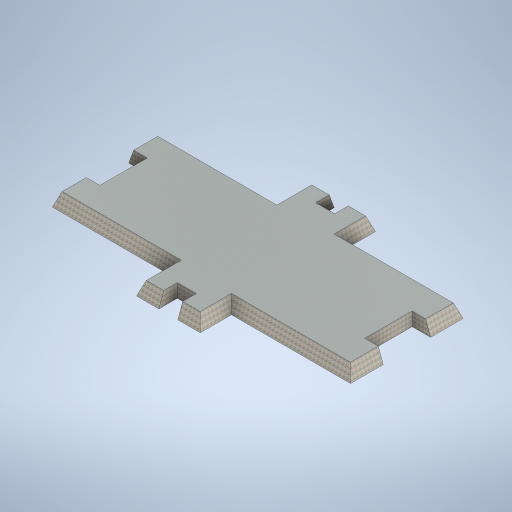
# Autodesk Inventor part: main_floor
Saved by Autodesk Inventor 2024.2 (Build 282272000, 272)
## iProperties
Created: 2024-05-24
Part Number: main_floor
Material: Limestone
Document SubType Name: Modeling
Designer: LOSTER_1
Density: 2.6 g/cm^3
Appearance: Limestone - Ashlar Coursed
Author: LOSTER_1
Autodesk Inventor part; units mm, degrees
ref_plane "YZ Plane" through (0, 0, 0) normal (1, 0, 0) x (0, 1, 0)
ref_plane "XZ Plane" through (0, 0, 0) normal (0, 1, 0) x (-1, 0, 0)
ref_plane "XY Plane" through (0, 0, 0) normal (0, 0, 1) x (1, 0, 0)
sketch "Sketch1" plane through (0, 0, 0) normal (0, 1, 0) x (-1, 0, 0)
  line L0 (-18589.1353, 7057.2083) -> (-18589.1353, -7090.0785)
  line L1 (18609.9901, -7090.0785) -> (18609.9901, 7057.2083)
  line L2 (18609.9901, 7057.2083) -> (21609.9901, 7057.2083)
  line L3 (21609.9901, 7057.2083) -> (21609.9901, -7090.0785)
  line L4 (21609.9901, -7090.0785) -> (18609.9901, -7090.0785)
  line L5 (18609.9901, -7090.0785) -> (18609.9901, 7057.2083)
  line L6 (-18589.1353, 7057.2083) -> (-21589.1353, 7057.2083)
  line L7 (-21589.1353, 7057.2083) -> (-21589.1353, -7090.0785)
  line L8 (-21589.1353, -7090.0785) -> (-18589.1353, -7090.0785)
  line L9 (-18589.1353, -7090.0785) -> (-18589.1353, 7057.2083)
  line L10 (18609.9901, 7057.2083) -> (3994.5778, 7057.2083)
  line L11 (-3973.723, 7057.2083) -> (-18589.1353, 7057.2083)
  line L12 (-18589.1353, -7090.0785) -> (-3973.723, -7090.0785)
  line L13 (3994.5778, -7090.0785) -> (18609.9901, -7090.0785)
  line L14 (3994.5778, -11251.4689) -> (3994.5778, -12251.4689)
  line L15 (3994.5778, -12251.4689) -> (1994.5778, -12251.4689)
  line L16 (-3973.723, 11218.7168) -> (-3973.723, 12218.7168)
  line L17 (-3973.723, 12218.7168) -> (-1973.723, 12218.7168)
  line L18 (3994.5778, -12251.4689) -> (-3973.723, -12251.4689)
  line L19 (-3973.723, -12251.4689) -> (-3973.723, 12218.7168)
  line L20 (-3973.723, 12218.7168) -> (3994.5778, 12218.7168)
  line L21 (3994.5778, 12218.7168) -> (3994.5778, -12251.4689)
  line L22 (21589.1353, 7600) -> (-21589.1353, 7600)
  line L23 (-21589.1353, 7600) -> (-21589.1353, -7600)
  line L24 (-21589.1353, -7600) -> (21589.1353, -7600)
  line L25 (21589.1353, 7600) -> (-21589.1353, -7600) construction
  line L26 (-21589.1353, 7600) -> (21589.1353, -7600) construction
  line L27 (10.4274, -12251.4689) -> (1410.4274, -12251.4689)
  line L28 (1410.4274, -12251.4689) -> (1410.4274, -10251.4689)
  line L29 (1410.4274, -10251.4689) -> (-1389.5726, -10251.4689)
  line L30 (-1389.5726, -10251.4689) -> (-1389.5726, -12251.4689)
  line L31 (10.4274, 12218.7168) -> (1410.4274, 12218.7168)
  line L32 (1410.4274, 12218.7168) -> (1410.4274, 10218.7168)
  line L33 (1410.4274, 10218.7168) -> (-1389.5726, 10218.7168)
  line L34 (-1389.5726, 10218.7168) -> (-1389.5726, 12218.7168)
  line L35 (-21589.1353, 0) -> (-19589.1353, 0)
  line L36 (-19589.1353, 0) -> (-21589.1353, 0)
  line L37 (-21589.1353, 0) -> (-21589.1353, 3500)
  line L38 (21589.1353, 7057.2083) -> (21589.1353, 7600)
  line L39 (21609.9901, -7090.0785) -> (21609.9901, -7600)
  line L40 (21589.1353, -7600) -> (21609.9901, -7600)
  line L41 (21609.9901, -16.4351) -> (21609.9901, -3516.4351)
  line L42 (21609.9901, -3516.4351) -> (19609.9901, -3516.4351)
  line L43 (19609.9901, -3516.4351) -> (19609.9901, 3483.5649)
  line L44 (19609.9901, 3483.5649) -> (21609.9901, 3483.5649)
  line L45 (21609.9901, 3483.5649) -> (21609.9901, -3516.4351)
  line L46 (-21589.1353, 3500) -> (-19589.1353, 3500)
  line L47 (-19589.1353, 3500) -> (-19589.1353, -3500)
  line L48 (-19589.1353, -3500) -> (-21589.1353, -3500)
  line L49 (-21589.1353, -3500) -> (-21589.1353, 3500)
  point P0 (1994.5778, 9218.7168)
  point P1 (1994.5778, -9251.4689)
  point P2 (-1973.723, -9251.4689)
  point P3 (-1973.723, -11251.4689)
  point P4 (0, 0)
  point P5 (3994.5778, -7600)
  point P6 (-3973.723, -7600)
  point P7 (-3973.723, 7600)
  point P8 (3994.5778, 7600)
  point P9 (21589.1353, -7090.0785)
  dimension "d0" = 3000
  dimension "d1" = 3000
  dimension "d12" = 15200
  dimension "d13" = 1400
  dimension "d14" = 2000
  dimension "d15" = 2800
  dimension "d16" = 1400
  dimension "d17" = 2000
  dimension "d18" = 2800
  dimension "d19" = 2000
  dimension "d21" = 3500
  dimension "d22" = 3500
  dimension "d23" = 2000
  dimension "d24" = 7000
  dimension "d27" = 2000
  dimension "d28" = 7000
  constraints: 100 end point, 17 parallel, 16 point on line, 12 perpendicular, 11 horizontal, 6 midpoint, 1 coincident, 1 vertical
  measures "d0" distance of L3.end L4.end
  measures "d1" distance of L8.end L7.end
  measures "d12" distance of L23.end L22.end
  measures "d13" distance of L27.start L27.end
  measures "d14" distance of L27.end L28.end
  measures "d15" distance of L28.end L29.end
  measures "d16" distance of L31.start L31.end
  measures "d17" distance of L31.end L32.end
  measures "d18" distance of L32.end L33.end
  measures "d19" distance of L35.start L35.end
  measures "d21" distance of L36.end L37.end
  measures "d22" distance of L41.start L41.end
  measures "d23" distance of L43.end L44.end
  measures "d24" distance of L42.end L43.end
  measures "d27" distance of L47.end L48.end
  measures "d28" distance of L46.end L47.end
extrude "Extrusion2" add sketch "Sketch1" against normal blind 2000 draft 20 contours L11 L19 L12 L0 | L0 L8 L7 L48 L47 L46 L6 | L6 L23 L22 L19 L11 | L12 L19 L24 L23 L8 | L19 L22 L21 L24 | L46 L47 L35 L7 | L19 L16 L17 L20 L34 L33 L32 L21 L22 | L7 L35 L47 L48 | L24 L21 L14 L15 L18 L28 L29 L30 L19 | L10 L1 L13 L21 | L30 L29 L28 L18 | L32 L33 L34 L20 | L2 L3 L44 L43 L42 L4 L1 | L3 L42 L43 L44
sketch "Sketch2" plane through (0, 0, 0) normal (0, 1, 0) x (1, 0, 0)
  line L0 (-1410.4274, -10218.7168) -> (1389.5726, -10218.7168) projected
  line L1 (-1410.4274, -10218.7168) -> (1389.5726, -10218.7168)
  line L2 (1389.5726, -10218.7168) -> (1389.5726, -19039.5456)
  line L3 (1389.5726, -19039.5456) -> (-1410.4274, -19039.5456)
  line L4 (-1410.4274, -19039.5456) -> (-1410.4274, -10218.7168)
  line L5 (-1410.4274, 10251.4689) -> (-1410.4274, 12251.4689) projected
  line L6 (-1410.4274, 10251.4689) -> (1389.5726, 10251.4689)
  line L7 (1389.5726, 10251.4689) -> (1389.5726, 17503.4785)
  line L8 (1389.5726, 17503.4785) -> (-1410.4274, 17503.4785)
  line L9 (-1410.4274, 17503.4785) -> (-1410.4274, 10251.4689)
  line L10 (-19609.9901, 3516.4351) -> (-19609.9901, -3483.5649) projected
  line L11 (-19609.9901, -3483.5649) -> (-29137.8877, -3483.5649)
  line L12 (-29137.8877, -3483.5649) -> (-29137.8877, 3516.4351)
  line L13 (-29137.8877, 3516.4351) -> (-19609.9901, 3516.4351)
  line L14 (-19609.9901, 3516.4351) -> (-19609.9901, -3483.5649)
  line L15 (19589.1353, 8.2175) -> (19589.1353, -3491.7825)
  line L16 (19589.1353, 8.2175) -> (19589.1353, 3508.2175)
  line L17 (19589.1353, -3491.7825) -> (31199.6373, -3491.7825)
  line L18 (31199.6373, -3491.7825) -> (31199.6373, 3508.2175)
  line L19 (31199.6373, 3508.2175) -> (19589.1353, 3508.2175)
  point P0 (0, 0)
  point P1 (19589.1353, -3500)
  dimension "d29" = 3500
  dimension "d30" = 3500
  constraints: 34 end point, 6 parallel, 5 perpendicular, 4 horizontal, 2 vertical, 1 point on line
  measures "d29" distance of L15.start L15.end
  measures "d30" distance of L15.start L16.end
extrude "Extrusion3" cut sketch "Sketch2" against normal blind 2000
sketch "Sketch3" plane through (0, 0, 0) normal (0, 1, 0) x (1, 0, 0)
  line L0 (1389.5726, -10218.7168) -> (-1410.4274, -10218.7168) projected
  line L1 (1389.5726, -12946.6572) -> (4701.6634, -12946.6572) projected
  line L2 (-1410.4274, -10218.7168) -> (1389.5726, -10218.7168)
  line L3 (1389.5726, -10218.7168) -> (1389.5726, -12946.6572)
  line L4 (1389.5726, -12946.6572) -> (-1410.4274, -12946.6572)
  line L5 (-1410.4274, -12946.6572) -> (-1410.4274, -10218.7168)
  point P0 (0, 0)
  constraints: 8 end point, 2 parallel, 1 horizontal, 1 perpendicular
body "Solid2"
